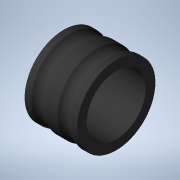
# Autodesk Inventor part: hpc_Q2307-ACC_2
Saved by Autodesk Inventor 2021 (Build 250183000, 183)
## iProperties
Created: 2026-05-26
Part Number: hpc_Q2307-ACC_2
Material: Generic
Catalog Web Link: www.3dfindit.com
Description: Q1Q2-2-Roulement à rotule sur billes - acier
Vendor: HPC
Document SubType Name: Modeling
Designer: psAdmin
Manufacturer: HPC
Mass: 20.2736 g
Surface Area: 93.882 cm^2
Volume: 20.2736 cm^3
Density: 1 g/cm^3
Appearance: PSOLRGB-176-176-176
Category: PARTsolutions
Company: HPC
Title: HPC - Q2307-ACC
Author: Cadenas PARTsolutions
Comments: Roulement à rotule sur billes - acier
PSOL_IDENT_0: {$CADENAS_DATA/23d-libs/hpc/v3/rotary/radial/steel/q1q2/q1q2_2.prj},171 {VTYP=3D},{NB=hpc_Q2307-ACC_
PSOL_IDENT_1: 2},{LINA=HPC - Q2307-ACC},{NN=Q1Q2-2},{DATE=26.05.2021 13:15:38},{GEOMDATE=24.09.2019 07:57:00},{VER
PSOL_IDENT_2: SION=},{LINEID=220},{WBVAR=},{WBNUMERIC=}  {NB=hpc_Q2307-ACC_2},{LINA=HPC - Q2307-ACC},{KT=DUMMY},{R
PSOL_IDENT_3: EF=Q2307-ACC},{D=35},{D1=80},{B=31},{CD=38.91},{CS=10.98},{VLG=9180},{VLH=10800},{MAS=0.680},{INFO=I
PSOL_IDENT_4: NFO}
NB: hpc_Q2307-ACC_2
NN: Q1Q2-2
NT: Roulement à rotule sur billes - acier
NBSYN: hpc_$REF._2
LINA: HPC - Q2307-ACC
CATALOG: HPC
REF: Q2307-ACC
D: 35
D1: 80
B: 31
CD: 38.91
CS: 10.98
VLG: 9180
VLH: 10800
MAS: 0.68
INFO: INFO
SUPPLIER: HPC
ARTICLENO: hpc_Q2307-ACC_2
BOMINFO: HPC - Q2307-ACC
CREATOR: CADENAS GmbH
Autodesk Inventor part; units mm, degrees
sketch "Sketch_1" plane through (0, 0, 0) normal (0, 0, 1) x (1, 0, 0)
  line L0 (50, 0) -> (-50, 0)
  line L1 (0, 23.1136) -> (0, 17.5)
  line L2 (0, 17.5) -> (31, 17.5)
  line L3 (31, 17.5) -> (31, 23.1136)
  line L4 (31, 23.1136) -> (27.7302, 23.1136)
  arc A0 (27.7302, 23.1136) -> (26.8226, 22.8599) centre (27.7302, 21.3636) ccw
  arc A1 (19.6774, 22.8599) -> (26.8226, 22.8599) centre (23.25, 28.75) ccw
  arc A2 (19.6774, 22.8599) -> (18.7698, 23.1136) centre (18.7698, 21.3636) ccw
  line L5 (18.7698, 23.1136) -> (12.2302, 23.1136)
  arc A3 (12.2302, 23.1136) -> (11.3226, 22.8599) centre (12.2302, 21.3636) ccw
  arc A4 (4.1774, 22.8599) -> (11.3226, 22.8599) centre (7.75, 28.75) ccw
  arc A5 (4.1774, 22.8599) -> (3.2698, 23.1136) centre (3.2698, 21.3636) ccw
  line L6 (3.2698, 23.1136) -> (0, 23.1136)
  constraints: 14 end point, 12 point on circle, 6 centre point
revolve "Revolution1" add sketch "Sketch_1" angle 360 about axis through (50, 0, 0) along (1, 0, 0)
ref_plane "IP_2_XY" through (15.5, 0, 0) normal (1, 0, 0) x (0, 0, -1)
ref_plane "IP_2_YZ" through (15.5, 0, 0) normal (0, 0, -1) x (0, 1, 0)
ref_plane "IP_2_ZX" through (15.5, 0, 0) normal (0, 1, 0) x (1, 0, 0)
ref_plane "IP_3_1_XY" through (7.75, 28.75, 0) normal (1, 0, 0) x (0, 0, -1)
ref_plane "IP_3_1_YZ" through (7.75, 28.75, 0) normal (0, 0, -1) x (0, 1, 0)
ref_plane "IP_3_1_ZX" through (7.75, 28.75, 0) normal (0, 1, 0) x (1, 0, 0)
ref_plane "IP_3_10_XY" through (7.75, 23.2592, -16.8988) normal (1, 0, 0) x (0, 0, -1)
ref_plane "IP_3_10_YZ" through (7.75, 23.2592, -16.8988) normal (0, 0, -1) x (0, 1, 0)
ref_plane "IP_3_10_ZX" through (7.75, 23.2592, -16.8988) normal (0, 1, 0) x (1, 0, 0)
ref_plane "IP_3_2_XY" through (7.75, 23.2592, 16.8988) normal (1, 0, 0) x (0, 0, -1)
ref_plane "IP_3_2_YZ" through (7.75, 23.2592, 16.8988) normal (0, 0, -1) x (0, 1, 0)
ref_plane "IP_3_2_ZX" through (7.75, 23.2592, 16.8988) normal (0, 1, 0) x (1, 0, 0)
ref_plane "IP_3_3_XY" through (7.75, 8.8842, 27.3429) normal (1, 0, 0) x (0, 0, -1)
ref_plane "IP_3_3_YZ" through (7.75, 8.8842, 27.3429) normal (0, 0, -1) x (0, 1, 0)
ref_plane "IP_3_3_ZX" through (7.75, 8.8842, 27.3429) normal (0, 1, 0) x (1, 0, 0)
ref_plane "IP_3_4_XY" through (7.75, -8.8842, 27.3429) normal (1, 0, 0) x (0, 0, -1)
ref_plane "IP_3_4_YZ" through (7.75, -8.8842, 27.3429) normal (0, 0, -1) x (0, 1, 0)
ref_plane "IP_3_4_ZX" through (7.75, -8.8842, 27.3429) normal (0, 1, 0) x (1, 0, 0)
ref_plane "IP_3_5_XY" through (7.75, -23.2592, 16.8988) normal (1, 0, 0) x (0, 0, -1)
ref_plane "IP_3_5_YZ" through (7.75, -23.2592, 16.8988) normal (0, 0, -1) x (0, 1, 0)
ref_plane "IP_3_5_ZX" through (7.75, -23.2592, 16.8988) normal (0, 1, 0) x (1, 0, 0)
ref_plane "IP_3_6_XY" through (7.75, -28.75, 0) normal (1, 0, 0) x (0, 0, -1)
ref_plane "IP_3_6_YZ" through (7.75, -28.75, 0) normal (0, 0, -1) x (0, 1, 0)
ref_plane "IP_3_6_ZX" through (7.75, -28.75, 0) normal (0, 1, 0) x (1, 0, 0)
ref_plane "IP_3_7_XY" through (7.75, -23.2592, -16.8988) normal (1, 0, 0) x (0, 0, -1)
ref_plane "IP_3_7_YZ" through (7.75, -23.2592, -16.8988) normal (0, 0, -1) x (0, 1, 0)
ref_plane "IP_3_7_ZX" through (7.75, -23.2592, -16.8988) normal (0, 1, 0) x (1, 0, 0)
ref_plane "IP_3_8_XY" through (7.75, -8.8842, -27.3429) normal (1, 0, 0) x (0, 0, -1)
ref_plane "IP_3_8_YZ" through (7.75, -8.8842, -27.3429) normal (0, 0, -1) x (0, 1, 0)
ref_plane "IP_3_8_ZX" through (7.75, -8.8842, -27.3429) normal (0, 1, 0) x (1, 0, 0)
ref_plane "IP_3_9_XY" through (7.75, 8.8842, -27.3429) normal (1, 0, 0) x (0, 0, -1)
ref_plane "IP_3_9_YZ" through (7.75, 8.8842, -27.3429) normal (0, 0, -1) x (0, 1, 0)
ref_plane "IP_3_9_ZX" through (7.75, 8.8842, -27.3429) normal (0, 1, 0) x (1, 0, 0)
ref_plane "IP_4_1_XY" through (23.25, 27.3429, 8.8842) normal (1, 0, 0) x (0, 0, -1)
ref_plane "IP_4_1_YZ" through (23.25, 27.3429, 8.8842) normal (0, 0, -1) x (0, 1, 0)
ref_plane "IP_4_1_ZX" through (23.25, 27.3429, 8.8842) normal (0, 1, 0) x (1, 0, 0)
ref_plane "IP_4_10_XY" through (23.25, 27.3429, -8.8842) normal (1, 0, 0) x (0, 0, -1)
ref_plane "IP_4_10_YZ" through (23.25, 27.3429, -8.8842) normal (0, 0, -1) x (0, 1, 0)
ref_plane "IP_4_10_ZX" through (23.25, 27.3429, -8.8842) normal (0, 1, 0) x (1, 0, 0)
ref_plane "IP_4_2_XY" through (23.25, 16.8988, 23.2592) normal (1, 0, 0) x (0, 0, -1)
ref_plane "IP_4_2_YZ" through (23.25, 16.8988, 23.2592) normal (0, 0, -1) x (0, 1, 0)
ref_plane "IP_4_2_ZX" through (23.25, 16.8988, 23.2592) normal (0, 1, 0) x (1, 0, 0)
ref_plane "IP_4_3_XY" through (23.25, 0, 28.75) normal (1, 0, 0) x (0, 0, -1)
ref_plane "IP_4_3_YZ" through (23.25, 0, 28.75) normal (0, 0, -1) x (0, 1, 0)
ref_plane "IP_4_3_ZX" through (23.25, 0, 28.75) normal (0, 1, 0) x (1, 0, 0)
ref_plane "IP_4_4_XY" through (23.25, -16.8988, 23.2592) normal (1, 0, 0) x (0, 0, -1)
ref_plane "IP_4_4_YZ" through (23.25, -16.8988, 23.2592) normal (0, 0, -1) x (0, 1, 0)
ref_plane "IP_4_4_ZX" through (23.25, -16.8988, 23.2592) normal (0, 1, 0) x (1, 0, 0)
ref_plane "IP_4_5_XY" through (23.25, -27.3429, 8.8842) normal (1, 0, 0) x (0, 0, -1)
ref_plane "IP_4_5_YZ" through (23.25, -27.3429, 8.8842) normal (0, 0, -1) x (0, 1, 0)
ref_plane "IP_4_5_ZX" through (23.25, -27.3429, 8.8842) normal (0, 1, 0) x (1, 0, 0)
ref_plane "IP_4_6_XY" through (23.25, -27.3429, -8.8842) normal (1, 0, 0) x (0, 0, -1)
ref_plane "IP_4_6_YZ" through (23.25, -27.3429, -8.8842) normal (0, 0, -1) x (0, 1, 0)
ref_plane "IP_4_6_ZX" through (23.25, -27.3429, -8.8842) normal (0, 1, 0) x (1, 0, 0)
ref_plane "IP_4_7_XY" through (23.25, -16.8988, -23.2592) normal (1, 0, 0) x (0, 0, -1)
ref_plane "IP_4_7_YZ" through (23.25, -16.8988, -23.2592) normal (0, 0, -1) x (0, 1, 0)
ref_plane "IP_4_7_ZX" through (23.25, -16.8988, -23.2592) normal (0, 1, 0) x (1, 0, 0)
ref_plane "IP_4_8_XY" through (23.25, 0, -28.75) normal (1, 0, 0) x (0, 0, -1)
ref_plane "IP_4_8_YZ" through (23.25, 0, -28.75) normal (0, 0, -1) x (0, 1, 0)
ref_plane "IP_4_8_ZX" through (23.25, 0, -28.75) normal (0, 1, 0) x (1, 0, 0)
ref_plane "IP_4_9_XY" through (23.25, 16.8988, -23.2592) normal (1, 0, 0) x (0, 0, -1)
ref_plane "IP_4_9_YZ" through (23.25, 16.8988, -23.2592) normal (0, 0, -1) x (0, 1, 0)
ref_plane "IP_4_9_ZX" through (23.25, 16.8988, -23.2592) normal (0, 1, 0) x (1, 0, 0)
body "Solid1"
